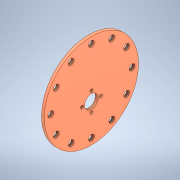
# Autodesk Inventor part: sample-transfer_plate
Saved by Autodesk Inventor 2020 (Build 240168000, 168)
## iProperties
Created: 2019-08-16
Part Number: sample-transfer_plate
Material: ABS Plastic orange
Document SubType Name: Modeling
Designer: rainer
Density: 1.06 g/cm^3
Appearance: Smooth - White
Author: rainer
Autodesk Inventor part; units mm, degrees
ref_plane "YZ Plane" through (0, 0, 0) normal (1, 0, 0) x (0, 1, 0)
ref_plane "XZ Plane" through (0, 0, 0) normal (0, 1, 0) x (-1, 0, 0)
ref_plane "XY Plane" through (0, 0, 0) normal (0, 0, 1) x (1, 0, 0)
sketch "Sketch1" plane through (0, 0, 0) normal (1, 0, 0) x (0, 1, 0)
  circle A0 centre (0, 0) radius 34.75
  circle A1 centre (-6.9, 0) radius 5
  dimension "d0" = 69.5
  dimension "d1" = 10
  dimension "d2" = 6.9
  constraints: 2 centre point, 1 coincident
  measures "d0" diameter of A0
  measures "d1" diameter of A1
  measures "d2" distance of point (0, 0) A1.centre
extrude "Extrusion1" add sketch "Sketch1" along normal blind 2
sketch "Sketch2" plane through (2, 0, 0) normal (1, 0, 0) x (0, 0, -1)
  circle A0 centre (0, 0) radius 30
  point P0 (0, 30)
  dimension "d5" = 60
  constraints: 1 coincident, 1 vertical alignment, 2 other
hole "Hole1" at (2, 30, 0) direction (-1, 0, 0) diameter 4.3 depth 10
pattern_circular "Circular Pattern1" count 12 over 360 about axis through (0, 0, 0) along (1, 0, 0) of "Hole1"
sketch "Sketch3" plane through (2, 0, 0) normal (1, 0, 0) x (0, 0, -1)
  circle A0 centre (0, -6.9) radius 5 projected
  circle A1 centre (0, -6.9) radius 7
  point P0 (0, 0)
  point P1 (0, 0.1)
  dimension "d16" = 14
  constraints: 1 coincident, 1 vertical alignment, 2 other
hole "Hole2" at (2, 0.1, 0) direction (-1, 0, 0) diameter 2.2 depth 10
pattern_circular "Circular Pattern2" count 4 over 360 about axis through (0, -6.9, 0) along (1, 0, 0) of "Hole2"
body "Solid1"
